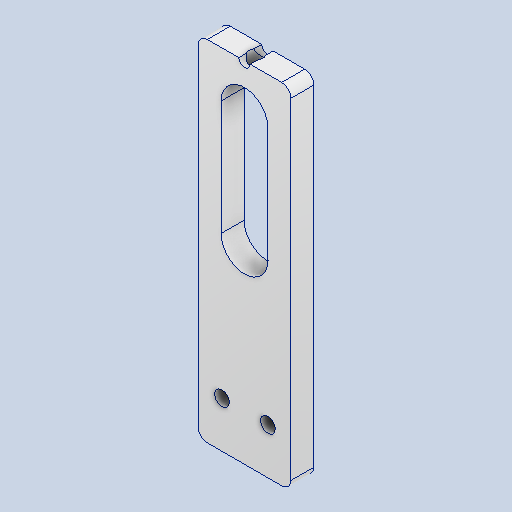
# Autodesk Inventor part: dribl-v3-Plate-16
Saved by Autodesk Inventor 2025.2 (Build 292293000, 293)
## iProperties
Created: 2025-04-09
Part Number: dribl-v3-Plate-16
Material: アルミニウム 6061
Document SubType Name: Modeling
Designer: haruy
Density: 2.7 g/cm^3
Appearance: アルミニウム - フラット
Author: haruy
Autodesk Inventor part; units mm, degrees
ref_plane "YZ Plane" through (0, 0, 0) normal (1, 0, 0) x (0, 1, 0)
ref_plane "XZ Plane" through (0, 0, 0) normal (0, 1, 0) x (-1, 0, 0)
ref_plane "XY Plane" through (0, 0, 0) normal (0, 0, 1) x (1, 0, 0)
derived "dribl-v3-Sketch-Base.ipt"
sketch "スケッチ5" plane through (-180, -184.3334, -303) normal (0, 0, 1) x (1, 0, 0)
  circle A0 centre (37.42, 41) radius 16 projected
  line L0 (0, -248) -> (0, 1189.5) projected
  line L1 (560, 20) -> (0, 20) projected
  circle A1 centre (10, 10) radius 1.6 projected
  circle A2 centre (30, 10) radius 1.6 projected
  line L2 (0, 0) -> (560, 0) projected
  line L3 (280, 20) -> (280, 0) projected
  circle A3 centre (522.58, 41) radius 16 projected
  circle A4 centre (530, 10) radius 1.6 projected
  circle A5 centre (550, 10) radius 1.6 projected
  circle A6 centre (-10, 10) radius 1.6 projected
  circle A7 centre (-10, -10) radius 1.6 projected
  line L4 (-20, 1189.5) -> (-20, -248) projected
  circle A8 centre (570, 10) radius 1.6 projected
  circle A9 centre (570, -10) radius 1.6 projected
  line L5 (420, 0) -> (420, 20) projected
  line L6 (560, -248) -> (560, 1189.5) projected
  line L7 (415, 20) -> (415, 0) projected
  circle A10 centre (404.9, 46) radius 16 projected
  circle A11 centre (404.9, 46) radius 5.1 projected
  line L8 (404.9, 46) -> (404.9, 0) projected
  line L9 (394.8, 20) -> (394.8, 0) projected
  circle A12 centre (404.9, 66) radius 5.1 projected
  circle A13 centre (404.9, 66) radius 10.1 projected
  line L10 (394.8, 20) -> (394.8, 66) projected
  line L11 (415, 20) -> (415, 66) projected
  line L12 (394.8, 66) -> (415, 66) projected
  line L13 (415, 66) -> (415, 76.1) projected
  line L14 (415, 76.1) -> (394.8, 76.1) projected
  line L15 (394.8, 76.1) -> (394.8, 66) projected
  line L16 (399.8, 46) -> (399.8, 66) projected
  line L17 (410, 66) -> (410, 46) projected
  circle A14 centre (410, 10) radius 1.6 projected
  circle A15 centre (400, 10) radius 1.6 projected
  line L18 (394.8, 0) -> (415, 0) projected
  line L19 (415, 0) -> (415, 20) projected
  line L20 (415, 20) -> (394.8, 20) projected
  line L21 (394.8, 20) -> (394.8, 0) projected
  circle A16 centre (404.9, 76.1) radius 1.25
  circle A17 centre (404.9, 41) radius 5.1 projected
  line L22 (399.8, 46) -> (399.8, 41) projected
  line L23 (410, 46) -> (410, 41) projected
  circle A18 centre (371.4, 45) radius 11 projected
  circle A19 centre (371.4, 45) radius 2 projected
  circle A20 centre (37.42, 41) radius 12.5 projected
  circle A21 centre (522.58, 41) radius 12.5 projected
  line L24 (522.58, 53.5) -> (37.42, 53.5) projected
  line L25 (37.42, 28.5) -> (522.58, 28.5) projected
  line L26 (360.4, 45) -> (360.4, 0) projected
  line L27 (382.4, 45) -> (382.4, 0) projected
  circle A22 centre (366.4, 10) radius 1.5 projected
  circle A23 centre (376.4, 10) radius 1.5 projected
  line L28 (449.4, 45) -> (449.4, 0) projected
  line L29 (427.4, 45) -> (427.4, 0) projected
  circle A24 centre (438.4, 45) radius 11 projected
  circle A25 centre (438.4, 45) radius 2 projected
  circle A26 centre (443.4, 10) radius 1.5 projected
  circle A27 centre (433.4, 10) radius 1.5 projected
  point P0 (180, 184.3334)
  point P1 (406.15, 76.1)
  point P2 (403.65, 76.1)
  dimension "d1" = 2.5
  constraints: 1 centre point, 1 midpoint, 1 point on circle
  measures "d1" diameter of A16
extrude "押し出し1" add sketch "スケッチ5" against normal blind 5 contours L25 L8 L1 L10 | L10 A10 L8 L25 | L10 A13 A10 | A10 A13 L16 L24 L10 | L10 L24 L16 L22 A17 L8 A10 | L1 L8 L2 L9 | L25 L11 L1 L8 | L8 A10 L11 L25 | A13 L12 L16 A10 | A10 L16 A13 | L15 L14 A16 A13 | A13 A16 L12 A12 | L8 A17 L23 L17 L24 L11 A10 | L1 L7 L2 L8 | L17 A13 A10 L11 L24 | L17 A10 A13 | A16 L14 L13 A13 | L12 A13 A10 L17 | A13 L11 A10
fillet "フィレット1" radius 2 4 edges at (214.8, -108.2334, -305.5) (235, -108.2334, -305.5) (235, -184.3334, -305.5) (214.8, -184.3334, -305.5)
sketch "スケッチ2" plane through (223.65, -108.2334, -303) normal (0, 1, 0) x (1, 0, 0)
  line L0 (-8.85, 5) -> (-8.85, 0) projected
  line L1 (2.5, 5) -> (9.35, 5) projected
  point P0 (-223.65, -303)
  point P1 (1.25, 2.5)
  dimension "d5" = 10.1
  dimension "d6" = 2.5
  measures "d5" distance from line of point (1.25, 2.5) L0
  measures "d6" distance from line of L1 point (1.25, 2.5)
hole "穴1" at (224.9, -108.2334, -305.5) direction (0, -1, 0) diameter 3 depth 10 tip angle 118
